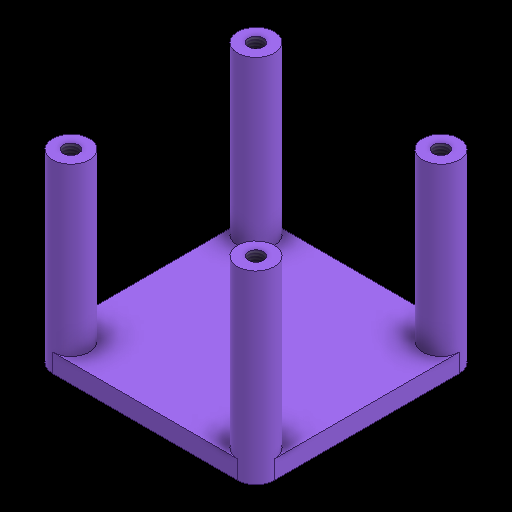
# Autodesk Inventor part: стойка для лотка
Saved by Autodesk Inventor 2025 (Build 290162000, 162)
## iProperties
Created: 2025-03-10
Part Number: стойка для лотка
Material: Типовые
Document SubType Name: Modeling
Designer: volko
Density: 1 g/cm^3
Appearance: Фиолетовый
Mass: 30.3747 g
Surface Area: 155.454 cm^2
Volume: 30.3747 cm^3
Author: volko
Autodesk Inventor part; units mm, degrees
ref_plane "YZ Plane" through (0, 0, 0) normal (1, 0, 0) x (0, 1, 0)
ref_plane "XZ Plane" through (0, 0, 0) normal (0, 1, 0) x (-1, 0, 0)
ref_plane "XY Plane" through (0, 0, 0) normal (0, 0, 1) x (1, 0, 0)
sketch "Эскиз1" plane through (0, 0, 0) normal (0, 1, 0) x (-1, 0, 0)
  line L0 (25, 30) -> (-25, 30)
  line L1 (-30, 25) -> (-30, -25)
  line L2 (-25, -30) -> (25, -30)
  line L3 (30, -25) -> (30, 25)
  line L4 (0, -43.4497) -> (0, 43.4497) projected
  line L5 (-43.4497, 0) -> (43.4497, 0) projected
  arc A0 (30, 25) -> (25, 30) centre (25, 25) ccw
  arc A1 (25, -30) -> (30, -25) centre (25, -25) ccw
  arc A2 (-30, -25) -> (-25, -30) centre (-25, -25) ccw
  arc A3 (-25, 30) -> (-30, 25) centre (-25, 25) ccw
  circle A4 centre (25, 25) radius 5
  circle A5 centre (25, -25) radius 5
  circle A6 centre (-25, 25) radius 5
  circle A7 centre (-25, -25) radius 5
  point P0 (0, 0)
  dimension "d0" = 5
  dimension "d1" = 25
  dimension "d2" = 25
  constraints: 8 centre point, 8 end point, 8 point on circle, 8 tangent, 4 equal radius, 3 symmetric about line, 2 parallel, 1 coincident, 1 horizontal, 1 perpendicular, 5 other
  measures "d0" radius of A0
  measures "d1" distance from line of L4 A0.centre
  measures "d2" distance from line of L5 A1.centre
extrude "Выдавливание1" add sketch "Эскиз1" along normal blind 5 contours A4 L3 L5 L4 L0 | L4 L5 L1 A6 L0 | L5 L3 A5 L2 L4 | L4 L2 A7 L1 L5
extrude "Выдавливание2" add sketch "Эскиз1" along normal blind 50 contours A0 A4 | A6 A3 | A1 A5 | A2 A7
hole "Отверстие1" at (25, 0, 25) at (-25, 0, 25) at (25, 0, -25) at (-25, 0, -25) direction (0, 1, 0) diameter 4.134 depth 15 tip angle 118 thread size "M5x0.8" class "6H" standard "ISO Metric profile"
sketch "Эскиз2" plane through (-25, 50, 25) normal (0, 1, 0) x (1, 0, 0)
  line L0 (-17, 25) -> (67, 25) projected
  line L1 (25, 67) -> (25, -17) projected
  point P0 (25, 25)
  point P1 (0.0023, -0.0231)
  point P2 (50.0023, -0.0231)
  point P3 (0.0023, 49.9769)
  point P4 (50.0023, 49.9769)
  dimension "d30" = 50
  dimension "d33" = 50
  constraints: 1 horizontal, 1 vertical, 3 other
  measures "d30" distance of point (0.002, -0.023) point (50.002, -0.023)
  measures "d33" distance of point (0.002, -0.023) point (0.002, 49.977)
hole "Отверстие3" at (-24.9977, 50, 25.0231) at (-24.9977, 50, -24.9769) at (25.0023, 50, -24.9769) at (25.0023, 50, 25.0231) direction (0, -1, 0) diameter 4.134 depth 15 tip angle 118 thread size "M5x0.8" class "6H" standard "ISO Metric profile"
